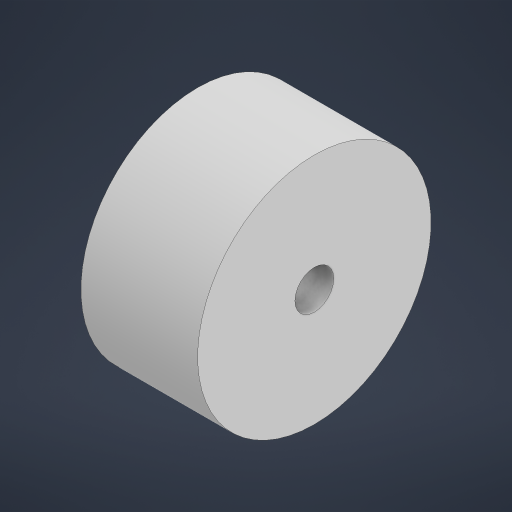
# Autodesk Inventor part: 30_diameter_wheel
Saved by Autodesk Inventor 2024 (Build 280153000, 153)
## iProperties
Created: 2023-06-18
Part Number: 30_diameter_wheel
Material: 일반
Document SubType Name: Modeling
Designer: 6gioc
Density: 1 g/cm^3
Appearance: 기본값
Author: 6gioc
Autodesk Inventor part; units mm, degrees
ref_plane "YZ Plane" through (0, 0, 0) normal (1, 0, 0) x (0, 1, 0)
ref_plane "XZ Plane" through (0, 0, 0) normal (0, 1, 0) x (-1, 0, 0)
ref_plane "XY Plane" through (0, 0, 0) normal (0, 0, 1) x (1, 0, 0)
sketch "스케치1" plane through (0, 0, 0) normal (1, 0, 0) x (0, 1, 0)
  circle A0 centre (0, 0) radius 2.5
  line L0 (2.5, 0) -> (2.1651, -1.25)
  line L1 (2.1651, -1.25) -> (1.25, -2.1651)
  line L2 (1.25, -2.1651) -> (0, -2.5)
  line L3 (0, -2.5) -> (-1.25, -2.1651)
  line L4 (-1.25, -2.1651) -> (-2.1651, -1.25)
  line L5 (-2.1651, -1.25) -> (-2.5, 0)
  line L6 (-2.5, 0) -> (-2.1651, 1.25)
  line L7 (-2.1651, 1.25) -> (-1.25, 2.1651)
  line L8 (-1.25, 2.1651) -> (0, 2.5)
  line L9 (0, 2.5) -> (1.25, 2.1651)
  line L10 (1.25, 2.1651) -> (2.1651, 1.25)
  line L11 (2.1651, 1.25) -> (2.5, 0)
  circle A1 centre (0, 0) radius 15
  dimension "d0" = 5
  dimension "d1" = 30
  constraints: 24 end point, 3 coincident, 1 centre point, 1 horizontal alignment, 27 other
  measures "d1" diameter of A1
extrude "돌출1" add sketch "스케치1" along normal blind 15
